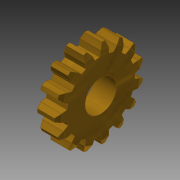
# Autodesk Inventor part: Zahnrad Messing z15
Saved by Autodesk Inventor 2017.3 (Build 213256000, 256)
## iProperties
Category: PARTsolutions
Company: MAEDLER
Created: 2018-08-20
Part Number: Zahnrad Messing z15
Material: Messing, weicher Gelbton, geschweißt
Catalog Web Link: www.cadenas.de
Description: Stzr Messing Ms58-Spur Gears, Brass, Helical Tooth Right Hand, with one-sided hub
Vendor: MAEDLER
Document SubType Name: Modeling
Designer: psadmin
Manufacturer: MAEDLER
Mass: 1.4 g
Surface Area: 2.77735 cm^2
Volume: 0.180679 cm^3
Density: 7.74853 g/cm^3
Appearance: Schweißnaht - Messing
PSOL_IDENT_0: {$CADENAS_DATA\23d-libs\maedler\antriebselemente\stirnzahnraeder\stirnzahnraeder_messing\stzr_messin
PSOL_IDENT_1: g_ms58.prj},204 {VTYP=3D},{NB=Stzr Messing Ms58 26101500},{LINA=Stzr Messing Ms58 26101500},{NN=Stzr
PSOL_IDENT_2: Messing Ms58},{DATE=03.08.2018 09:08:56},{GEOMDATE=26.07.2018 09:15:44},{VERSION=},{LINEID=220},{WB
PSOL_IDENT_3: VAR=},{WBNUMERIC=}  {NB=Stzr Messing Ms58 26101500},{LINA=Stzr Messing Ms58 26101500},{KT=DUMMY},{AR
PSOL_IDENT_4: TNR=26101500},{WST=Messing (Ms58)},{M=0.5},{Z=15},{PDF=PDF Katalogseite},{B1=2.0},{DA=8.50},{D=7.50}
PSOL_IDENT_5: ,{NL=4},{ND=6},{B=2.00},{MD=0.8},{GEW=1.400}
NN: Stzr Messing Ms58
NT: Spur Gears, Brass, Helical Tooth Right Hand, with one-sided hub
NB: Stzr Messing Ms58 26101500
NBSYN: Stzr Messing Ms58 $ARTNR.
LINA: Stzr Messing Ms58 26101500
ARTNR: 26101500
WST: Messing (Ms58)
M: 0.5
Z: 15
PDF: PDF Katalogseite
B1: 2
DA: 8.5
D: 7.5
NL: 4
ND: 6
B: 2
MD: 0.8
GEW: 1.4
SUPPLIER: MAEDLER
ARTICLENO: Stzr Messing Ms58 26101500
BOMINFO: Stzr Messing Ms58 26101500
CREATOR: CADENAS GmbH
Title: Stzr Messing Ms58 26101500
Author: Cadenas PARTsolutions
Comments: Spur Gears, Brass, Helical Tooth Right Hand, with one-sided hub
Autodesk Inventor part; units mm, degrees
ref_plane "YZ Plane" through (0, 0, 0) normal (1, 0, 0) x (0, 1, 0)
ref_plane "XZ Plane" through (0, 0, 0) normal (0, 1, 0) x (-1, 0, 0)
ref_plane "XY Plane" through (0, 0, 0) normal (0, 0, 1) x (1, 0, 0)
sketch "Skizze_1" plane through (0, 0, 0) normal (0, 0, 1) x (1, 0, 0)
  line L0 (6, 0) -> (0, 0)
  line L1 (0, 1) -> (6, 1)
  line L2 (6, 1) -> (6, 3)
  line L3 (6, 3) -> (2, 3)
  line L4 (2, 3) -> (2, 3.75)
  line L5 (2, 3.75) -> (1, 6.4975)
  line L6 (1, 6.4975) -> (0, 3.75)
  line L7 (0, 3.75) -> (0, 1)
  constraints: 16 end point
revolve "Revolution1" add sketch "Skizze_1" angle 360 about axis through (6, 0, 0) along (1, 0, 0)
sketch "Skizze_2" plane through (2, 0, 0) normal (1, 0, 0) x (0, 0, -1)
  circle A0 centre (0, 0) radius 12.75
  line L0 (-4.2409, 0.2782) -> (-3.75, 0.0117)
  line L1 (-3.75, 0.0117) -> (-3.248, -0.1134)
  arc A1 (-3.248, -0.1134) -> (-3.2006, -0.5644) centre (0, 0) ccw
  line L2 (-3.2006, -0.5644) -> (-3.6656, -0.7911)
  line L3 (-3.6656, -0.7911) -> (-4.0904, -1.1538)
  arc A2 (-4.0904, -1.1538) -> (-3.9874, -1.4708) centre (0, 0) ccw
  line L4 (-3.9874, -1.4708) -> (-3.4305, -1.5145)
  line L5 (-3.4305, -1.5145) -> (-2.9211, -1.4247)
  arc A3 (-2.9211, -1.4247) -> (-2.6944, -1.8174) centre (0, 0) ccw
  line L6 (-2.6944, -1.8174) -> (-3.0269, -2.2137)
  line L7 (-3.0269, -2.2137) -> (-3.2675, -2.7178)
  arc A4 (-3.2675, -2.7178) -> (-3.0444, -2.9655) centre (0, 0) ccw
  line L8 (-3.0444, -2.9655) -> (-2.5179, -2.7789)
  line L9 (-2.5179, -2.7789) -> (-2.0891, -2.4896)
  arc A5 (-2.0891, -2.4896) -> (-1.7222, -2.7562) centre (0, 0) ccw
  line L10 (-1.7222, -2.7562) -> (-1.8648, -3.2534)
  line L11 (-1.8648, -3.2534) -> (-1.8796, -3.8118)
  arc A6 (-1.8796, -3.8118) -> (-1.575, -3.9474) centre (0, 0) ccw
  line L12 (-1.575, -3.9474) -> (-1.17, -3.5628)
  line L13 (-1.17, -3.5628) -> (-0.8958, -3.1241)
  arc A7 (-0.8958, -3.1241) -> (-0.4523, -3.2184) centre (0, 0) ccw
  line L14 (-0.4523, -3.2184) -> (-0.3803, -3.7307)
  line L15 (-0.3803, -3.7307) -> (-0.1667, -4.2467)
  arc A8 (-0.1667, -4.2467) -> (0.1667, -4.2467) centre (0, 0) ccw
  line L16 (0.1667, -4.2467) -> (0.3803, -3.7307)
  line L17 (0.3803, -3.7307) -> (0.4523, -3.2184)
  arc A9 (0.4523, -3.2184) -> (0.8958, -3.1241) centre (0, 0) ccw
  line L18 (0.8958, -3.1241) -> (1.17, -3.5628)
  line L19 (1.17, -3.5628) -> (1.575, -3.9474)
  arc A10 (1.575, -3.9474) -> (1.8796, -3.8118) centre (0, 0) ccw
  line L20 (1.8796, -3.8118) -> (1.8648, -3.2534)
  line L21 (1.8648, -3.2534) -> (1.7222, -2.7562)
  arc A11 (1.7222, -2.7562) -> (2.0891, -2.4896) centre (0, 0) ccw
  line L22 (2.0891, -2.4896) -> (2.5179, -2.7789)
  line L23 (2.5179, -2.7789) -> (3.0444, -2.9655)
  arc A12 (3.0444, -2.9655) -> (3.2675, -2.7178) centre (0, 0) ccw
  line L24 (3.2675, -2.7178) -> (3.0269, -2.2137)
  line L25 (3.0269, -2.2137) -> (2.6944, -1.8174)
  arc A13 (2.6944, -1.8174) -> (2.9211, -1.4247) centre (0, 0) ccw
  line L26 (2.9211, -1.4247) -> (3.4305, -1.5145)
  line L27 (3.4305, -1.5145) -> (3.9874, -1.4708)
  arc A14 (3.9874, -1.4708) -> (4.0904, -1.1538) centre (0, 0) ccw
  line L28 (4.0904, -1.1538) -> (3.6656, -0.7911)
  line L29 (3.6656, -0.7911) -> (3.2006, -0.5644)
  arc A15 (3.2006, -0.5644) -> (3.248, -0.1134) centre (0, 0) ccw
  line L30 (3.248, -0.1134) -> (3.75, 0.0117)
  line L31 (3.75, 0.0117) -> (4.2409, 0.2782)
  arc A16 (4.2409, 0.2782) -> (4.206, 0.6097) centre (0, 0) ccw
  line L32 (4.206, 0.6097) -> (3.6705, 0.7682)
  line L33 (3.6705, 0.7682) -> (3.1535, 0.7862)
  arc A17 (3.1535, 0.7862) -> (3.0133, 1.2175) centre (0, 0) ccw
  line L34 (3.0133, 1.2175) -> (3.421, 1.536)
  line L35 (3.421, 1.536) -> (3.7611, 1.979)
  arc A18 (3.7611, 1.979) -> (3.5944, 2.2677) centre (0, 0) ccw
  line L36 (3.5944, 2.2677) -> (3.0407, 2.1947)
  line L37 (3.0407, 2.1947) -> (2.561, 2.0009)
  arc A19 (2.561, 2.0009) -> (2.2576, 2.3379) centre (0, 0) ccw
  line L38 (2.2576, 2.3379) -> (2.5005, 2.7946)
  line L39 (2.5005, 2.7946) -> (2.631, 3.3377)
  arc A20 (2.631, 3.3377) -> (2.3613, 3.5336) centre (0, 0) ccw
  line L40 (2.3613, 3.5336) -> (1.8851, 3.2417)
  line L41 (1.8851, 3.2417) -> (1.5258, 2.8696)
  arc A21 (1.5258, 2.8696) -> (1.1116, 3.054) centre (0, 0) ccw
  line L42 (1.1116, 3.054) -> (1.1477, 3.5701)
  line L43 (1.1477, 3.5701) -> (1.046, 4.1193)
  arc A22 (1.046, 4.1193) -> (0.7199, 4.1886) centre (0, 0) ccw
  line L44 (0.7199, 4.1886) -> (0.4036, 3.7282)
  line L45 (0.4036, 3.7282) -> (0.2267, 3.2421)
  arc A23 (0.2267, 3.2421) -> (-0.2267, 3.2421) centre (0, 0) ccw
  line L46 (-0.2267, 3.2421) -> (-0.4036, 3.7282)
  line L47 (-0.4036, 3.7282) -> (-0.7199, 4.1886)
  arc A24 (-0.7199, 4.1886) -> (-1.046, 4.1193) centre (0, 0) ccw
  line L48 (-1.046, 4.1193) -> (-1.1477, 3.5701)
  line L49 (-1.1477, 3.5701) -> (-1.1116, 3.054)
  arc A25 (-1.1116, 3.054) -> (-1.5258, 2.8696) centre (0, 0) ccw
  line L50 (-1.5258, 2.8696) -> (-1.8851, 3.2417)
  line L51 (-1.8851, 3.2417) -> (-2.3613, 3.5336)
  arc A26 (-2.3613, 3.5336) -> (-2.631, 3.3377) centre (0, 0) ccw
  line L52 (-2.631, 3.3377) -> (-2.5005, 2.7946)
  line L53 (-2.5005, 2.7946) -> (-2.2576, 2.3379)
  arc A27 (-2.2576, 2.3379) -> (-2.561, 2.0009) centre (0, 0) ccw
  line L54 (-2.561, 2.0009) -> (-3.0407, 2.1947)
  line L55 (-3.0407, 2.1947) -> (-3.5944, 2.2677)
  arc A28 (-3.5944, 2.2677) -> (-3.7611, 1.979) centre (0, 0) ccw
  line L56 (-3.7611, 1.979) -> (-3.421, 1.536)
  line L57 (-3.421, 1.536) -> (-3.0133, 1.2175)
  arc A29 (-3.0133, 1.2175) -> (-3.1535, 0.7862) centre (0, 0) ccw
  line L58 (-3.1535, 0.7862) -> (-3.6705, 0.7682)
  line L59 (-3.6705, 0.7682) -> (-4.206, 0.6097)
  arc A30 (-4.206, 0.6097) -> (-4.2409, 0.2782) centre (0, 0) ccw
  constraints: 120 end point, 60 point on circle, 31 centre point
extrude "Extrusion1" cut sketch "Skizze_2" along normal mid plane 12
sketch "Skizze3" plane through (0, 0, 0) normal (-1, 0, 0) x (0, 0, 1)
  point P0 (0, 0)
  point P1 (0, 0)
  constraints: 1 coincident
hole "Bohrung1" at (0, 0, 0) direction (1, 0, 0) diameter 3 end through all
sketch "Skizze4" plane through (6, 0, 0) normal (1, 0, 0) x (0, 0, -1)
  circle A0 centre (0, 0) radius 3 projected
extrude "Extrusion2" cut sketch "Skizze4" against normal blind 4
body "Solid1"
